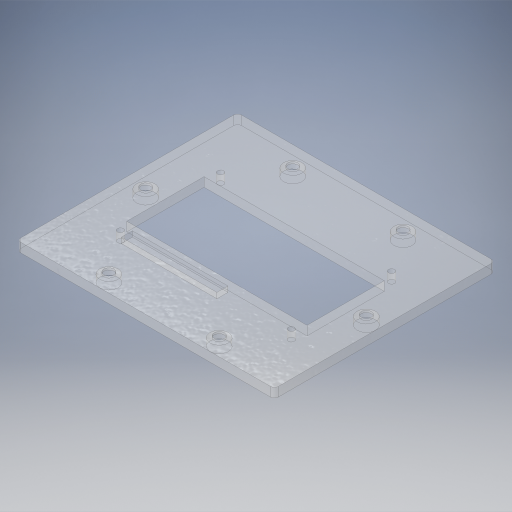
# Autodesk Inventor part: BT701_trajan20_21
Saved by Autodesk Inventor 2023 (Build 270158000, 158)
## iProperties
Company: HTBLA Kaindorf
RuleStatus: InUse
Created: 2022-08-21
Part Number: BT701_trajan20_21
Project: Zeichenmaschine_v2
Material: Acryl
Description: Plexi_100x80
Document SubType Name: Modeling
Designer: trajan20
Density: 1.188 g/cm^3
Appearance: Transparent - farblos
Mass: 71.5987 g
Surface Area: 304.034 cm^2
Volume: 60.2683 cm^3
AfterDocNew0: iProperties-Editor_aufrufen
Author: jan
Keywords: 2021
Autodesk Inventor part; units mm, degrees
ref_plane "YZ Plane" through (0, 0, 0) normal (1, 0, 0) x (0, 1, 0)
ref_plane "XZ Plane" through (0, 0, 0) normal (0, 1, 0) x (-1, 0, 0)
ref_plane "XY Plane" through (0, 0, 0) normal (0, 0, 1) x (1, 0, 0)
derived "BT000_trajan20_22_Zeichenmaschine_neu_Masterskizze.ipt"
sketch "Skizze3" plane through (0, 0, 0) normal (0, 0, 1) x (1, 0, 0)
  line L0 (0, 0) -> (-120, 0)
  line L1 (-120, 0) -> (-120, 140)
  line L2 (-120, 140) -> (0, 140)
  line L3 (0, 140) -> (0, 0)
  line L4 (-120, 140) -> (0, 140)
  line L5 (-32.75, 23.5) -> (-87.25, 23.5) construction
  line L6 (-87.25, 23.5) -> (-87.25, 116.5) construction
  line L7 (-89.75, 21) -> (-29.75, 21)
  line L8 (-29.75, 21) -> (-29.75, 119)
  line L9 (-29.75, 119) -> (-89.75, 119)
  line L10 (-89.75, 119) -> (-89.75, 21)
  line L11 (-29.75, 113) -> (-35.75, 113) construction
  line L12 (-29.75, 67) -> (-35.75, 67) construction
  line L13 (-35.75, 67) -> (-35.75, 113) construction
  line L14 (-38.75, 119) -> (-38.75, 21)
  line L15 (-80.75, 119) -> (-80.75, 21)
  line L16 (-29.75, 27) -> (-35.75, 27)
  line L17 (-35.75, 27) -> (-35.75, 79)
  line L18 (-29.75, 79) -> (-35.75, 79)
  point P0 (-10, 40)
  point P1 (-10, 100)
  point P2 (-110, 40)
  point P3 (-110, 100)
  point P4 (-60, 10)
  point P5 (-60, 130)
  point P6 (-60, 140)
  point P7 (-32.75, 116.5)
  point P8 (-60, 23.5)
  point P9 (-60, 0)
  point P10 (-87.25, 70)
  point P11 (-120, 70)
  dimension "d4" = 140
  dimension "d5" = 120
  dimension "d19" = 10
  dimension "d20" = 10
  dimension "d21" = 10
  dimension "d22" = 10
  dimension "d23" = 40
  dimension "d24" = 40
  dimension "d33" = 93
  dimension "d34" = 54.5
  dimension "d35" = 98
  dimension "d36" = 60
  dimension "d37" = 2.5
  dimension "d38" = 2.5
  dimension "d39" = 6
  dimension "d40" = 52
  dimension "d41" = 6
  dimension "d42" = 9
  dimension "d43" = 9
  dimension "d55" = 6
  dimension "d56" = 52
  constraints: 38 end point, 9 point on line, 8 perpendicular, 7 vertical alignment, 6 horizontal, 5 horizontal alignment, 5 midpoint, 5 parallel
  measures "d4" distance between parallel lines of L2 L0
  measures "d5" distance between parallel lines of L1 L3
  measures "d19" distance from line of L3 point (-10, 40)
  measures "d20" distance from line of L1 point (-110, 40)
  measures "d21" distance from line of L0 point (-60, 10)
  measures "d22" distance from line of L2 point (-60, 130)
  measures "d23" distance from line of L2 point (-110, 100)
  measures "d24" distance from line of L0 point (-110, 40)
  measures "d33" distance of L6.end L5.end
  measures "d34" distance of L5.end L5.start
  measures "d35" distance of L7.end L8.end
  measures "d36" distance of L8.end L9.end
  measures "d37" distance from line of L10 L5.end
  measures "d38" distance from line of L7 L5.end
  measures "d39" distance between parallel lines of L9 L11
  measures "d40" distance between parallel lines of L12 L9
  measures "d41" distance between parallel lines of L13 L8
  measures "d42" distance between parallel lines of L15 L10
  measures "d43" distance between parallel lines of L8 L14
  measures "d55" distance between parallel lines of L7 L16
  measures "d56" distance between parallel lines of L16 L18
extrude "Extrusion3" add sketch "Skizze3" along normal blind 5 contours L0 L1 L2 L3 | L10 L9 L15 L7 | L15 L9 L14 L7 | L14 L9 L8 L18 L17 L16 L7 | L16 L17 L18 L8
fillet "Rundung3" radius 2 4 edges at (0, 0, 2.5) (0, 140, 2.5) (-120, 140, 2.5) (-120, 0, 2.5)
hole "Bohrung1" at (-10, 40, 0) at (-10, 100, 0) at (-110, 40, 0) at (-110, 100, 0) at (-60, 10, 0) at (-60, 130, 0) direction (0, 0, 1) diameter 5.5 end through all counterbore diameter 10 counterbore depth 4
sketch "Skizze5" plane through (0, 0, 5) normal (0, 0, 1) x (1, 0, 0)
  circle A0 centre (-60, 10) radius 2.75 projected
  circle A1 centre (-110, 40) radius 2.75 projected
  circle A2 centre (-10, 40) radius 2.75 projected
  circle A3 centre (-10, 100) radius 2.75 projected
  circle A4 centre (-110, 100) radius 2.75 projected
  circle A5 centre (-60, 130) radius 2.75 projected
  arc A6 (-120, 2) -> (-118, 0) centre (-118, 2) ccw projected
  line L0 (-118, 0) -> (-2, 0) projected
  arc A7 (-2, 0) -> (0, 2) centre (-2, 2) ccw projected
  line L1 (0, 2) -> (0, 138) projected
  arc A8 (0, 138) -> (-2, 140) centre (-2, 138) ccw projected
  line L2 (-2, 140) -> (-118, 140) projected
  arc A9 (-118, 140) -> (-120, 138) centre (-118, 138) ccw projected
  line L3 (-120, 138) -> (-120, 2) projected
  line L4 (-29.75, 79) -> (-35.75, 79) projected
  line L5 (-35.75, 67) -> (-35.75, 113) construction
  line L6 (-35.75, 27) -> (-35.75, 79) projected
  line L7 (-29.75, 21) -> (-29.75, 119) projected
  line L8 (-29.75, 27) -> (-35.75, 27) projected
  point P0 (0, 0)
extrude "Extrusion6" cut sketch "Skizze5" against normal blind 3 contours L7 L8 L6 L4
extrude "Extrusion7" cut sketch "Skizze3" along normal blind 10 contours L15 L9 L14 L7
hole "Bohrung2" at (-87.25, 23.5, 0) at (-87.25, 116.5, 0) at (-32.75, 23.5, 0) at (-32.75, 116.5, 0) direction (0, 0, 1) diameter 3.3 end through all
equation "\"d4\" = Basis_Haupt_Breite_Profillänge + 4 * AluProfil_Abstand"
equation "\"d5\" = Basis_Haupt_Höhe_Profillänge"
equation "\"d19\" = AluProfil_Abstand"
equation "\"d20\" = AluProfil_Abstand"
equation "\"d21\" = AluProfil_Abstand"
equation "\"d22\" = AluProfil_Abstand"
equation "\"d24\" = d23"
equation "\"d55\" = d39"
equation "\"d56\" = d40"
equation "\"Basis_Haupt_Breite_Profillänge\" = 100"
equation "\"AluProfil_Abstand\" = 10"
equation "\"Basis_Haupt_Höhe_Profillänge\" = 120"
